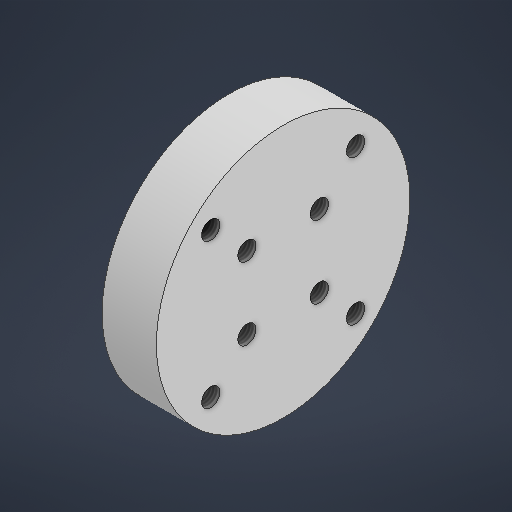
# Autodesk Inventor part: EndEffectorThreadedSupport
Saved by Autodesk Inventor 2025 (Build 290162000, 162)
## iProperties
Created: 2024-05-20
Part Number: EndEffectorThreadedSupport
Material: Generic
Document SubType Name: Modeling
Designer: avsar
Density: 1 g/cm^3
Appearance: Default
Author: avsar
Autodesk Inventor part; units mm, degrees
ref_plane "YZ Plane" through (0, 0, 0) normal (1, 0, 0) x (0, 1, 0)
ref_plane "XZ Plane" through (0, 0, 0) normal (0, 1, 0) x (-1, 0, 0)
ref_plane "XY Plane" through (0, 0, 0) normal (0, 0, 1) x (1, 0, 0)
sketch "Sketch1" plane through (0, 0, 0) normal (1, 0, 0) x (0, 1, 0)
  circle A0 centre (0, 0) radius 16 construction
  circle A1 centre (8, 8) radius 2
  circle A2 centre (-8, 8) radius 2
  circle A3 centre (-8, -8) radius 2
  circle A4 centre (8, -8) radius 2
  circle A5 centre (0, 0) radius 28
  circle A6 centre (16, 16) radius 2
  line L0 (0, 0) -> (0, -16) construction
  circle A7 centre (-16, 16) radius 2
  line L1 (0, 0) -> (-16, 0) construction
  circle A8 centre (16, -16) radius 2
  circle A9 centre (-16, -16) radius 2
  dimension "d0" = 32
  dimension "d1" = 4
  dimension "d2" = 8
  dimension "d3" = 8
  dimension "d6" = 360
  dimension "d8" = 56
  dimension "d9" = 4
  dimension "d10" = 16
  dimension "d11" = 16
  constraints: 10 centre point, 4 end point, 3 symmetric about line, 2 coincident, 2 point on circle, 1 horizontal, 1 vertical, 12 other
  measures "d0" diameter of A0
  measures "d1" diameter of A1
  measures "d2" horizontal distance of point (0, 0) A1.centre
  measures "d3" horizontal distance of point (0, 0) A1.centre
  measures "d8" diameter of A5
  measures "d9" diameter of A6
  measures "d10" horizontal distance of point (0, 0) A6.centre
  measures "d11" horizontal distance of point (0, 0) A6.centre
extrude "Extrusion1" add sketch "Sketch1" along normal blind 12
thread "Thread1" size "M4x0.7" class "6H" standard "ANSI Metric M Profile" full length
thread "Thread2" size "M4x0.7" class "6H" standard "ANSI Metric M Profile" full length
thread "Thread3" size "M4x0.7" class "6H" standard "ANSI Metric M Profile" full length
thread "Thread4" size "M4x0.7" class "6H" standard "ANSI Metric M Profile" full length
thread "Thread5" size "M4x0.7" class "6H" standard "ANSI Metric M Profile" full length
thread "Thread6" size "M4x0.7" class "6H" standard "ANSI Metric M Profile" full length
thread "Thread7" size "M4x0.7" class "6H" standard "ANSI Metric M Profile" full length
thread "Thread8" size "M4x0.7" class "6H" standard "ANSI Metric M Profile" full length
body "Solid1"
